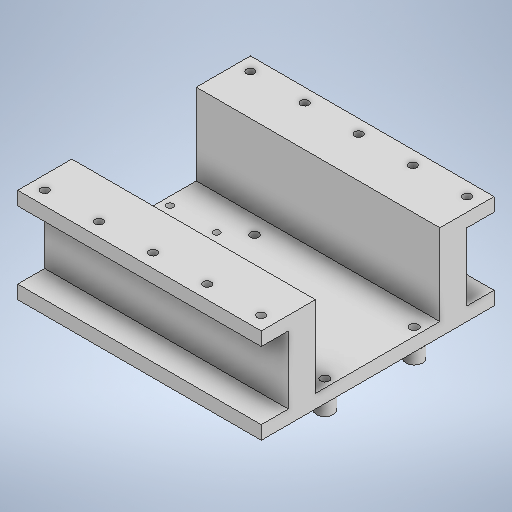
# Autodesk Inventor part: Battery_zig
Saved by Autodesk Inventor 2025 (Build 290162010, 162A)
## iProperties
Created: 2024-09-12
Part Number: Battery_zig
Material: Generic
Document SubType Name: Modeling
Designer: fist5
Density: 1 g/cm^3
Appearance: Default
Author: fist5
Autodesk Inventor part; units mm, degrees
ref_plane "YZ Plane" through (0, 0, 0) normal (1, 0, 0) x (0, 1, 0)
ref_plane "XZ Plane" through (0, 0, 0) normal (0, 1, 0) x (-1, 0, 0)
ref_plane "XY Plane" through (0, 0, 0) normal (0, 0, 1) x (1, 0, 0)
sketch "Sketch1" plane through (0, 0, 0) normal (0, 1, 0) x (-1, 0, 0)
  line L0 (45, -43) -> (-45, -43)
  line L1 (-45, -43) -> (-45, 43)
  line L2 (-45, 43) -> (45, 43)
  line L3 (45, 43) -> (45, -43)
  line L4 (45, -43) -> (-45, 43) construction
  line L5 (-45, -43) -> (45, 43) construction
  point P0 (0, 0)
  dimension "d0" = 90
  dimension "d1" = 86
  constraints: 12 end point, 2 midpoint, 2 parallel, 1 horizontal, 1 perpendicular
  measures "d0" distance between parallel lines of L1 L3
  measures "d1" distance between parallel lines of L2 L0
extrude "Extrusion1" add sketch "Sketch1" along normal blind 5
sketch "Sketch2" plane through (0, 5, 0) normal (0, 1, 0) x (1, 0, 0)
  line L0 (-45, 43) -> (-45, -43) projected
  line L1 (45, -43) -> (45, 43) projected
  line L2 (-45, 33) -> (45, 33)
  line L3 (45, 33) -> (45, 23)
  line L4 (45, 23) -> (-45, 23)
  line L5 (-45, 23) -> (-45, 33)
  line L6 (-45, -23) -> (45, -23)
  line L7 (45, -23) -> (45, -33)
  line L8 (45, -33) -> (-45, -33)
  line L9 (-45, -33) -> (-45, -23)
  point P0 (0, 0)
  point P1 (45, 0)
  point P2 (-45, -33)
  point P3 (45, -23)
  point P4 (-45, 23)
  point P5 (45, 33)
  dimension "d4" = 46
  dimension "d5" = 23
  dimension "d6" = 10
  dimension "d7" = 10
  constraints: 16 end point, 4 parallel, 4 point on line, 2 horizontal, 2 perpendicular, 1 horizontal alignment, 1 midpoint
  measures "d4" distance between parallel lines of L6 L4
  measures "d5" distance of L3.end point (45, 0)
  measures "d6" distance between parallel lines of L4 L2
  measures "d7" distance between parallel lines of L8 L6
extrude "Extrusion2" add sketch "Sketch2" along normal blind 30 contours L2 L1 L4 L0 | L6 L1 L8 L0
sketch "Sketch3" plane through (45, 5, -33) normal (0, 0, -1) x (-1, 0, 0)
  line L0 (0, 0) -> (0, 30) projected
  line L1 (90, 0) -> (90, 30) projected
  line L2 (0, 30) -> (90, 30)
  line L3 (90, 30) -> (90, 25)
  line L4 (90, 25) -> (0, 25)
  line L5 (0, 25) -> (0, 30)
  point P0 (45, -5)
  point P1 (0, 25)
  dimension "d10" = 5
  constraints: 8 end point, 2 parallel, 1 horizontal, 1 perpendicular, 1 point on line
  measures "d10" distance between parallel lines of L2 L4
extrude "Extrusion3" add sketch "Sketch3" along normal blind 10
sketch "Sketch4" plane through (-45, 5, 33) normal (0, 0, 1) x (1, 0, 0)
  line L0 (90, 0) -> (90, 25) projected
  line L1 (0, 30) -> (90, 30)
  line L2 (90, 30) -> (90, 25)
  line L3 (90, 25) -> (0, 25)
  line L4 (0, 25) -> (0, 30)
  point P0 (45, -5)
  constraints: 8 end point, 2 parallel, 1 horizontal, 1 perpendicular
extrude "Extrusion4" add sketch "Sketch4" along normal blind 10
sketch "Sketch5" plane through (0, 35, 0) normal (0, 1, 0) x (1, 0, 0)
  circle A0 centre (40, 38) radius 1.5
  line L0 (-45, 43) -> (45, 43) projected
  line L1 (45, 23) -> (45, 43) projected
  circle A1 centre (40, -38) radius 1.5
  circle A2 centre (20, 38) radius 1.5
  circle A3 centre (20, -38) radius 1.5
  circle A4 centre (0, 38) radius 1.5
  circle A5 centre (0, -38) radius 1.5
  circle A6 centre (-20, 38) radius 1.5
  circle A7 centre (-20, -38) radius 1.5
  circle A8 centre (-40, 38) radius 1.5
  circle A9 centre (-40, -38) radius 1.5
  point P0 (0, 0)
  dimension "d15" = 3
  dimension "d21" = 5
  dimension "d22" = 5
  dimension "d25" = 76
  dimension "d28" = 20
  constraints: 10 centre point, 1 horizontal, 1 vertical, 18 other
  measures "d15" diameter of A0
  measures "d21" distance from line of L0 A0.centre
  measures "d22" distance from line of L1 A0.centre
  measures "d25" distance of A0.centre A1.centre
  measures "d28" distance of A0.centre A2.centre
extrude "Extrusion5" cut sketch "Sketch5" against normal up to surface (5 mm away)
sketch "Sketch6" plane through (0, 0, 0) normal (0, -1, 0) x (1, 0, 0)
  line L0 (42, 16.5) -> (-17, 16.5)
  line L1 (-17, 16.5) -> (-17, -16.5)
  line L2 (-17, -16.5) -> (42, -16.5)
  line L3 (42, -16.5) -> (42, 16.5)
  line L4 (42, 16.5) -> (-17, -16.5) construction
  line L5 (-17, 16.5) -> (42, -16.5) construction
  line L6 (-42, 10.25) -> (-24.75, 10.25)
  line L7 (-24.75, 10.25) -> (-24.75, -10.25)
  line L8 (-24.75, -10.25) -> (-42, -10.25)
  line L9 (-42, -10.25) -> (-42, 10.25)
  line L10 (-42, 10.25) -> (-24.75, -10.25) construction
  line L11 (-24.75, 10.25) -> (-42, -10.25) construction
  circle A0 centre (-24.75, 10.25) radius 1.25
  circle A1 centre (-24.75, -10.25) radius 1.25
  circle A2 centre (-42, 10.25) radius 1.25
  circle A3 centre (-42, -10.25) radius 1.25
  line L12 (-45, -43) -> (-45, 43) projected
  line L13 (45, 43) -> (45, -43) projected
  circle A4 centre (42, 16.5) radius 1.6
  circle A5 centre (-17, 16.5) radius 1.6
  circle A6 centre (-17, -16.5) radius 1.6
  circle A7 centre (42, -16.5) radius 1.6
  point P0 (0, 0)
  point P1 (12.5, 0)
  point P2 (-33.375, 0)
  point P3 (-33.375, -10.25)
  point P4 (-33.375, 10.25)
  dimension "d35" = 33
  dimension "d36" = 59
  dimension "d37" = 20.5
  dimension "d38" = 17.25
  dimension "d39" = 2.5
  dimension "d42" = 20.5
  dimension "d45" = 17.25
  dimension "d48" = 3
  dimension "d49" = 3
  dimension "d50" = 3.2
  dimension "d51" = 3.2
  dimension "d52" = 3.2
  dimension "d53" = 3.2
  constraints: 24 end point, 8 centre point, 6 midpoint, 5 coincident, 4 parallel, 3 horizontal, 2 horizontal alignment, 2 perpendicular, 1 vertical, 6 other
  measures "d35" distance between parallel lines of L2 L0
  measures "d36" distance between parallel lines of L1 L3
  measures "d37" distance of point (-33.375, -10.25) point (-33.375, 10.25)
  measures "d38" distance between parallel lines of L9 L7
  measures "d39" diameter of A0
  measures "d42" distance of A0.centre A1.centre
  measures "d45" distance of A0.centre A2.centre
  measures "d48" distance between parallel lines of L12 L9
  measures "d49" distance between parallel lines of L13 L3
  measures "d50" diameter of A5
  measures "d51" diameter of A6
  measures "d52" diameter of A7
  measures "d53" diameter of A4
extrude "Extrusion6" cut sketch "Sketch6" against normal up to surface (5 mm away) contours A5 L1 L0 | L0 L1 A5 | A4 L3 L0 | L0 L3 A4 | A6 L2 L1 | L1 L2 A6 | A7 L2 L3 | L3 L2 A7 | L9 A2 L6 | L6 A2 L9 | A0 L7 L6 | L6 L7 A0 | A3 L8 L9 | L9 L8 A3 | A1 L8 L7 | L7 L8 A1
sketch "Sketch7" plane through (0, 0, 0) normal (0, -1, 0) x (1, 0, 0)
  circle A0 centre (-17, -16.5) radius 1.6 projected
  circle A1 centre (42, 16.5) radius 1.6 projected
  circle A2 centre (-24.75, 10.25) radius 1.25 projected
  circle A3 centre (-42, 10.25) radius 1.25 projected
  circle A4 centre (-17, 16.5) radius 1.6 projected
  circle A5 centre (42, -16.5) radius 1.6 projected
  circle A6 centre (-24.75, -10.25) radius 1.25 projected
  circle A7 centre (-42, -10.25) radius 1.25 projected
  line L0 (-45, 43) -> (45, 43) projected
  line L1 (-45, -43) -> (-45, 43) projected
  line L2 (45, -43) -> (-45, -43) projected
  line L3 (45, 43) -> (45, -43) projected
  circle A8 centre (42, 16.5) radius 3.1
  circle A9 centre (42, -16.5) radius 3.1
  circle A10 centre (-17, -16.5) radius 3.1
  circle A11 centre (-24.75, -10.25) radius 2.75
  circle A12 centre (-17, 16.5) radius 3.1
  circle A13 centre (-24.75, 10.25) radius 2.75
  circle A14 centre (-42, 10.25) radius 2.75
  circle A15 centre (-42, -10.25) radius 2.75
  point P0 (0, 0)
  dimension "d56" = 1.5
  dimension "d57" = 1.5
  dimension "d58" = 1.5
  dimension "d59" = 1.5
  dimension "d60" = 1.5
  dimension "d61" = 1.5
  dimension "d62" = 1.5
  dimension "d63" = 1.5
  constraints: 8 centre point, 8 coincident
  measures "d56" radial gap between concentric circles of A8 A1
  measures "d57" radial gap between concentric circles of A9 A5
  measures "d58" radial gap between concentric circles of A10 A0
  measures "d59" radial gap between concentric circles of A11 A6
  measures "d60" radial gap between concentric circles of A15 A7
  measures "d61" radial gap between concentric circles of A14 A3
  measures "d62" radial gap between concentric circles of A13 A2
  measures "d63" radial gap between concentric circles of A12 A4
extrude "Extrusion7" add sketch "Sketch7" along normal blind 5 contours A8 L3 | L3 A8 | A9 L3 | L3 A9 | A10 | A11 | A12 | A13 | A14 | A15
body "Solid1"
